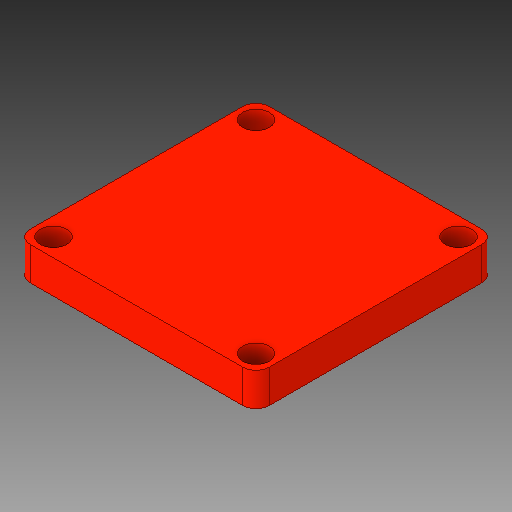
# Autodesk Inventor part: Flight_controler
Saved by Autodesk Inventor 2018 (Build 220112000, 112)
## iProperties
Created: 2017-12-31
Part Number: Flight_controler
Material: Generic
Document SubType Name: Modeling
Designer: suchanek
Density: 1 g/cm^3
Appearance: Default
Mass: 6.2115 g
Surface Area: 34.3876 cm^2
Volume: 6.2115 cm^3
Author: suchanek
Autodesk Inventor part; units mm, degrees
ref_plane "YZ Plane" through (0, 0, 0) normal (1, 0, 0) x (0, 1, 0)
ref_plane "XZ Plane" through (0, 0, 0) normal (0, 1, 0) x (-1, 0, 0)
ref_plane "XY Plane" through (0, 0, 0) normal (0, 0, 1) x (1, 0, 0)
sketch "Sketch1" plane through (0, 0, 0) normal (0, 1, 0) x (-1, 0, 0)
  line L0 (0, 0) -> (18, 0)
  line L1 (16, -18) -> (-16, -18)
  line L2 (-18, -16) -> (-18, 16)
  line L3 (-16, 18) -> (16, 18)
  line L4 (18, 16) -> (18, -16)
  circle A0 centre (15.25, 15.25) radius 2
  circle A1 centre (-15.25, 15.25) radius 2
  circle A2 centre (-15.25, -15.25) radius 2
  circle A3 centre (15.25, -15.25) radius 2
  arc A4 (16, -18) -> (18, -16) centre (16, -16) ccw
  arc A5 (18, 16) -> (16, 18) centre (16, 16) ccw
  arc A6 (-16, 18) -> (-18, 16) centre (-16, 16) ccw
  arc A7 (-18, -16) -> (-16, -18) centre (-16, -16) ccw
  point P0 (18, -18)
  point P1 (-18, 18)
  point P2 (-18, -18)
  point P3 (18, 18)
  dimension "d0" = 18
  dimension "d1" = 18
  dimension "d2" = 36
  dimension "d3" = 36
  dimension "d6" = 30.5
  dimension "d7" = 30.5
  dimension "d8" = 15.25
  dimension "d9" = 2.75
  dimension "d10" = 4
  dimension "d11" = 4
  dimension "d12" = 4
  dimension "d13" = 4
  dimension "d14" = 2
  dimension "d15" = 2
  constraints: 10 end point, 8 centre point, 8 point on circle, 8 point on line, 8 tangent, 3 vertical alignment, 2 equal radius, 2 horizontal, 2 horizontal alignment, 2 parallel, 1 perpendicular
  measures "d0" distance of L0.start L0.end
  measures "d1" distance of L0.end point (18, -18)
  measures "d2" distance of point (-18, 18) point (18, 18)
  measures "d3" distance of point (-18, -18) point (-18, 18)
  measures "d6" distance of A3.centre A0.centre
  measures "d7" distance of A1.centre A0.centre
  measures "d8" distance from line of L0 A0.centre
  measures "d9" distance from line of L4 A0.centre
  measures "d10" diameter of A0
  measures "d11" diameter of A1
  measures "d12" diameter of A2
  measures "d13" diameter of A3
  measures "d14" radius of A4
  measures "d15" radius of A5
extrude "Extrusion2" add sketch "Sketch1" along normal blind 5
body "Solid2"
